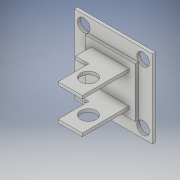
# Autodesk Inventor part: pneumatics back holder
Saved by Autodesk Inventor 2018 (Build 220112000, 112)
## iProperties
Created: 2019-01-16
Part Number: pneumatics back holder
Material: Generic
Document SubType Name: Modeling
Designer: s-4008082
Density: 1 g/cm^3
Appearance: Default
Author: s-4008082
Autodesk Inventor part; units mm, degrees
ref_plane "YZ Plane" through (0, 0, 0) normal (1, 0, 0) x (0, 1, 0)
ref_plane "XZ Plane" through (0, 0, 0) normal (0, 1, 0) x (-1, 0, 0)
ref_plane "XY Plane" through (0, 0, 0) normal (0, 0, 1) x (1, 0, 0)
sketch "Sketch1" plane through (0, 0, 0) normal (0, 0, 1) x (1, 0, 0)
  line L0 (15.875, 15.875) -> (-15.875, 15.875)
  line L1 (-15.875, 15.875) -> (-15.875, -15.875)
  line L2 (-15.875, -15.875) -> (15.875, -15.875)
  line L3 (15.875, -15.875) -> (15.875, 15.875)
  line L4 (15.875, 15.875) -> (-15.875, -15.875) construction
  line L5 (-15.875, 15.875) -> (15.875, -15.875) construction
  point P0 (0, 0)
  dimension "d0" = 31.75
  dimension "d1" = 31.75
  constraints: 12 end point, 2 midpoint, 2 parallel, 1 horizontal, 1 perpendicular
  measures "d0" distance of L0.start L0.end
  measures "d1" distance of L2.end L0.start
extrude "Extrusion1" add sketch "Sketch1" along normal blind 1.27
sketch "Sketch2" plane through (0, 0, 1.27) normal (0, 0, 1) x (1, 0, 0)
  line L0 (-10.16, 10.16) -> (10.16, 10.16)
  line L1 (10.16, 10.16) -> (10.16, -10.16)
  line L2 (10.16, -10.16) -> (-10.16, -10.16)
  line L3 (-10.16, -10.16) -> (-10.16, 10.16)
  line L4 (15.875, 15.875) -> (-15.875, 15.875) projected
  line L5 (15.875, -15.875) -> (15.875, 15.875) projected
  line L6 (-15.875, -15.875) -> (15.875, -15.875) projected
  line L7 (-15.875, 15.875) -> (-15.875, -15.875) projected
  point P0 (0, 0)
  dimension "d4" = 5.715
  dimension "d5" = 5.715
  dimension "d6" = 5.715
  dimension "d7" = 5.715
  constraints: 8 end point, 2 parallel, 1 horizontal, 1 perpendicular
  measures "d4" distance between parallel lines of L4 L0
  measures "d5" distance between parallel lines of L5 L1
  measures "d6" distance between parallel lines of L6 L2
  measures "d7" distance between parallel lines of L7 L3
extrude "Extrusion2" add sketch "Sketch2" along normal blind 1.27 contours L0 L1 L2 L3
sketch "Sketch3" plane through (0, 0, 2.54) normal (0, 0, 1) x (1, 0, 0)
  line L0 (-7.62, 5.9817) -> (7.62, 5.9817)
  line L1 (7.62, 5.9817) -> (7.62, 7.2517)
  line L2 (7.62, 7.2517) -> (-7.62, 7.2517)
  line L3 (-7.62, 7.2517) -> (-7.62, 5.9817)
  line L4 (10.16, -10.16) -> (10.16, 10.16) projected
  line L5 (-10.16, 10.16) -> (-10.16, -10.16) projected
  line L6 (10.16, 10.16) -> (-10.16, 10.16) projected
  line L7 (-7.62, -7.2517) -> (7.62, -7.2517)
  line L8 (7.62, -7.2517) -> (7.62, -5.9817)
  line L9 (7.62, -5.9817) -> (-7.62, -5.9817)
  line L10 (-7.62, -5.9817) -> (-7.62, -7.2517)
  line L11 (-10.16, -10.16) -> (10.16, -10.16) projected
  point P0 (0, 0)
  dimension "d48" = 1.27
  dimension "d49" = 11.9634
  dimension "d50" = 1.27
  dimension "d54" = 2.54
  dimension "d55" = 2.54
  dimension "d56" = 2.54
  dimension "d57" = 2.54
  dimension "d58" = 2.9083
  dimension "d59" = 2.921
  constraints: 16 end point, 4 parallel, 2 horizontal, 2 perpendicular
  measures "d48" distance of L7.end L8.end
  measures "d49" distance between parallel lines of L9 L0
  measures "d50" distance of L0.end L1.end
  measures "d54" distance between parallel lines of L5 L3
  measures "d55" distance between parallel lines of L4 L1
  measures "d56" distance between parallel lines of L5 L10
  measures "d57" distance between parallel lines of L4 L8
  measures "d58" distance between parallel lines of L11 L7
extrude "Extrusion3" add sketch "Sketch3" along normal blind 19.05 contours L3 L2 L1 L0 | L10 L9 L8 L7
sketch "Sketch4" plane through (-7.62, -7.2517, 2.54) normal (0, -1, 0) x (1, 0, 0)
  circle A0 centre (10.16, 11.43) radius 3.175
  line L0 (0, 19.05) -> (15.24, 19.05) projected
  line L1 (0, 0) -> (0, 19.05) projected
  point P0 (7.62, -2.54)
  dimension "d20" = 6.35
  dimension "d21" = 7.62
  dimension "d44" = 10.16
  constraints: 1 centre point
  measures "d20" diameter of A0
  measures "d21" distance from line of L0 A0.centre
  measures "d44" distance from line of L1 A0.centre
extrude "Extrusion4" cut sketch "Sketch4" against normal blind 127
sketch "Sketch5" plane through (0, 0, 1.27) normal (0, 0, 1) x (1, 0, 0)
  circle A0 centre (-12.065, 12.065) radius 2.5797
  line L0 (-15.875, -15.875) -> (15.875, -15.875) projected
  line L1 (15.875, -15.875) -> (15.875, 15.875) projected
  circle A1 centre (12.065, 12.065) radius 2.5797
  line L2 (15.875, 15.875) -> (-15.875, 15.875) projected
  line L3 (-15.875, 15.875) -> (-15.875, -15.875) projected
  circle A2 centre (-12.065, -12.065) radius 2.5797
  circle A3 centre (12.065, -12.065) radius 2.5797
  point P0 (0, 0)
  dimension "d24" = 5.1594
  dimension "d28" = 5.1594
  dimension "d29" = 3.81
  dimension "d30" = 3.81
  dimension "d31" = 3.81
  dimension "d32" = 3.81
  dimension "d33" = 5.1594
  dimension "d34" = 3.81
  dimension "d35" = 3.81
  dimension "d36" = 5.1594
  dimension "d37" = 3.81
  dimension "d38" = 3.81
  constraints: 4 centre point
  measures "d24" diameter of A0
  measures "d28" diameter of A1
  measures "d29" distance from line of L2 A0.centre
  measures "d30" distance from line of L3 A0.centre
  measures "d31" distance from line of L2 A1.centre
  measures "d32" distance from line of L1 A1.centre
  measures "d33" diameter of A2
  measures "d34" distance from line of L3 A2.centre
  measures "d35" distance from line of L0 A2.centre
  measures "d36" diameter of A3
  measures "d37" distance from line of L0 A3.centre
  measures "d38" distance from line of L1 A3.centre
extrude "Extrusion5" cut sketch "Sketch5" against normal blind 12.7 contours A0 | A1 | A2 | A3
sketch "Sketch6" plane through (-7.62, -7.2517, 2.54) normal (0, -1, 0) x (1, 0, 0)
  line L0 (0, 0) -> (0, 19.05) projected
  line L1 (0, 19.05) -> (15.24, 19.05) projected
  line L2 (0, 6.5528) -> (5.4184, 6.5528)
  line L3 (5.4184, 6.5528) -> (5.4184, 19.05)
  line L4 (5.4184, 19.05) -> (0, 19.05)
  line L5 (0, 19.05) -> (0, 6.5528)
  point P0 (7.62, -2.54)
  constraints: 8 end point, 2 parallel, 2 point on line, 1 horizontal, 1 perpendicular
extrude "Extrusion6" cut sketch "Sketch6" against normal blind 101.6
equation "\"d5\" = d4"
equation "\"d6\" = d4"
equation "\"d7\" = d4"
equation "\"d50\" = d48"
equation "\"d55\" = d54"
equation "\"d56\" = d54"
equation "\"d57\" = d54"
equation "\"d28\" = d24"
equation "\"d30\" = d29"
equation "\"d31\" = d29"
equation "\"d32\" = d29"
equation "\"d33\" = d24"
equation "\"d34\" = d29"
equation "\"d35\" = d29"
equation "\"d36\" = d24"
equation "\"d37\" = d29"
equation "\"d38\" = d29"
body "Solid1"
